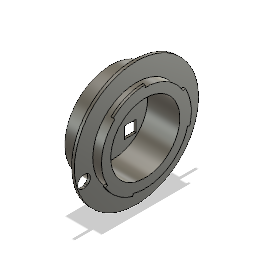
mft_multi_pinhole_lens (Autodesk Fusion 360 design; units mm, degrees)
Autodesk Fusion 360 part; units mm, degrees
sketch "スケッチ1" plane through (0, 0, 0) normal (1, 0, 0) x (0, 0, -1)
  circle A0 centre (0, 0) radius 27
  dimension "d1" = 54
  measures "d1" diameter of A0
extrude "押し出し1" add sketch "スケッチ1" along normal blind 1.2
sketch "スケッチ2" plane through (1.2, 0, 0) normal (1, 0, 0) x (0, 0, -1)
  circle A0 centre (0, 0) radius 27
  circle A1 centre (0, 0) radius 19
  dimension "d4" = 38
  measures "d4" diameter of A1
extrude "押し出し2" add sketch "スケッチ2" along normal blind 3.8 contours A1
sketch "スケッチ7" plane through (5, 0, 0) normal (1, 0, 0) x (0, 0, -1)
  circle A0 centre (0, 0) radius 19
  arc A1 (0, 20) -> (-13.9054, 14.375) centre (0, 0) ccw
  arc A2 (-17.3011, -10.0336) -> (-5.4591, -19.2405) centre (0, 0) ccw
  arc A3 (19.3599, -5.0193) -> (17.3316, 9.9807) centre (0, 0) ccw
  line L0 (17.3316, 9.9807) -> (0, 0)
  line L1 (0, 0) -> (19.3599, -5.0193)
  line L2 (0, 20) -> (0, 0)
  line L3 (-13.9054, 14.375) -> (0, 0)
  line L4 (-17.3011, -10.0336) -> (0, 0)
  line L5 (-5.4591, -19.2405) -> (0, 0)
  dimension "d10" = 20
  dimension "d11" = 20
  dimension "d12" = 20
  dimension "d13" = 15
  dimension "d14" = 15
  dimension "d15" = 15
  measures "d10" radius of A1
  measures "d11" radius of A2
  measures "d12" radius of A3
  measures "d14" distance of A0.centre
extrude "押し出し3" add sketch "スケッチ7" against normal blind 1 contours A0 A3 L0 L1 | A0 A1 L2 L3 | A0 A2 L4 L5
sketch "スケッチ12" plane through (1.2, 0, 0) normal (1, 0, 0) x (0, 0, -1)
  circle A0 centre (0, 0) radius 19
  circle A1 centre (0, 0) radius 27
  arc A2 (-24.592, -5.0724) -> (-22.0631, -9.3178) centre (-23, -7) ccw
  arc A3 (-21.3514, -8.9648) -> (-23.2882, -4.3834) centre (-22.5544, -6.7733) ccw
  line L0 (-22.0631, -9.3178) -> (-21.3514, -8.9648)
  line L1 (-24.592, -5.0724) -> (-23.2882, -4.3834)
  dimension "d38" = 2.5
  dimension "d39" = 2.5
  dimension "d62" = 0.5
  dimension "d63" = 1.476
  measures "d38" radius of A2
  measures "d39" radius of A3
  measures "d63" angle of L0 L1
extrude "押し出し10" cut sketch "スケッチ12" against normal blind 11 contours A2 A3 L0 L1
sketch "スケッチ8" plane through (0, 0, 0) normal (-1, 0, 0) x (0, 0, 1)
  circle A0 centre (0, 0) radius 27
  circle A1 centre (0, 0) radius 20
  arc A2 (23.2882, -4.3834) -> (21.3514, -8.9648) centre (22.5544, -6.7733) ccw
  line L0 (23.2882, -4.3834) -> (24.592, -5.0724)
  arc A3 (22.0631, -9.3178) -> (24.592, -5.0724) centre (23, -7) ccw
  line L1 (22.0631, -9.3178) -> (21.3514, -8.9648)
  dimension "d18" = 40
  measures "d18" diameter of A1
extrude "押し出し4" add sketch "スケッチ8" along normal blind 10 contours A1
sketch "スケッチ9" plane through (5, 0, 0) normal (1, 0, 0) x (0, 0, -1)
  arc A0 (16.465, 9.4817) -> (0, 19) centre (0, 0) ccw
  line L0 (0, 19) -> (0, 20)
  arc A1 (0, 20) -> (-13.9054, 14.375) centre (0, 0) ccw
  line L1 (-13.9054, 14.375) -> (-13.2101, 13.6563)
  arc A2 (-13.2101, 13.6563) -> (-16.436, -9.5319) centre (0, 0) ccw
  line L2 (-16.436, -9.5319) -> (-17.3011, -10.0336)
  arc A3 (-17.3011, -10.0336) -> (-5.4591, -19.2405) centre (0, 0) ccw
  line L3 (-5.4591, -19.2405) -> (-5.1861, -18.2785)
  arc A4 (-5.1861, -18.2785) -> (18.3919, -4.7683) centre (0, 0) ccw
  line L4 (18.3919, -4.7683) -> (19.3599, -5.0193)
  arc A5 (19.3599, -5.0193) -> (17.3316, 9.9807) centre (0, 0) ccw
  line L5 (17.3316, 9.9807) -> (16.465, 9.4817)
  circle A6 centre (0, 0) radius 15
  dimension "d21" = 30
  measures "d21" diameter of A6
extrude "押し出し5" cut sketch "スケッチ9" against normal blind 14 contours A6
sketch "スケッチ11" plane through (-9, 0, 0) normal (1, 0, 0) x (0, 0, -1)
  circle A0 centre (0, 0) radius 15
  line L0 (-2.5, 2.5) -> (2.5, 2.5)
  line L1 (2.5, 2.5) -> (2.5, -2.5)
  line L2 (2.5, -2.5) -> (-2.5, -2.5)
  line L3 (-2.5, -2.5) -> (-2.5, 2.5)
  line L4 (5, 10) -> (10, 10)
  line L5 (10, 10) -> (10, 5)
  line L6 (10, 5) -> (5, 5)
  line L7 (5, 5) -> (5, 10)
  line L8 (-10, 10) -> (-5, 10)
  line L9 (-5, 10) -> (-5, 5)
  line L10 (-5, 5) -> (-10, 5)
  line L11 (-10, 5) -> (-10, 10)
  line L12 (-10, -5) -> (-5, -5)
  line L13 (-5, -5) -> (-5, -10)
  line L14 (-5, -10) -> (-10, -10)
  line L15 (-10, -10) -> (-10, -5)
  line L16 (5, -5) -> (10, -5)
  line L17 (10, -5) -> (10, -10)
  line L18 (10, -10) -> (5, -10)
  line L19 (5, -10) -> (5, -5)
  dimension "d42" = 5
  dimension "d43" = 2.5
  dimension "d44" = 2.5
  dimension "d45" = 5
  dimension "d46" = 5
  dimension "d47" = 5
  dimension "d48" = 5
  dimension "d49" = 5
  dimension "d50" = 5
  dimension "d51" = 5
  dimension "d52" = 5
  dimension "d53" = 5
  dimension "d54" = 5
  dimension "d55" = 5
  dimension "d56" = 5
  dimension "d57" = 5
  dimension "d58" = 5
  dimension "d59" = 5
  measures "d43" distance of A0.centre L1
  measures "d44" distance of A0.centre L0
  measures "d47" distance of A0.centre L6
  measures "d48" distance of A0.centre L7
  measures "d51" distance of A0.centre L10
  measures "d52" distance of A0.centre L9
  measures "d53" distance of A0.centre L13
  measures "d54" distance of A0.centre L19
  measures "d59" distance of A0.centre L12
extrude "押し出し11" cut sketch "スケッチ11" against normal blind 5 contours L0 L1 L2 L3 | L4 L5 L6 L7 | L8 L9 L10 L11 | L12 L13 L14 L15 | L16 L17 L18 L19
